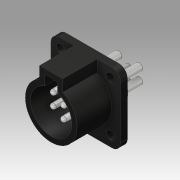
# Autodesk Inventor part: 6pin
Saved by Autodesk Inventor 2019.3 (Build 233278000, 278)
## iProperties
Created: 2019-05-28
Part Number: 6pin
Material: Generic
Document SubType Name: Modeling
Designer: Dave
Density: 1 g/cm^3
Appearance: Default
Author: Dave
Autodesk Inventor part; units mm, degrees
ref_plane "YZ Plane" through (0, 0, 0) normal (1, 0, 0) x (0, 1, 0)
ref_plane "XZ Plane" through (0, 0, 0) normal (0, 1, 0) x (-1, 0, 0)
ref_plane "XY Plane" through (0, 0, 0) normal (0, 0, 1) x (1, 0, 0)
sketch "Sketch1" plane through (0, 0, 0) normal (0, 0, 1) x (1, 0, 0)
  line L0 (2.5, 0) -> (17.7, 0)
  line L1 (20.2, 2.5) -> (20.2, 17.7)
  line L2 (17.7, 20.2) -> (2.5, 20.2)
  line L3 (0, 17.7) -> (0, 2.5)
  circle A0 centre (2.85, 17.35) radius 1.25
  circle A1 centre (17.35, 17.35) radius 1.25
  circle A2 centre (17.35, 2.85) radius 1.25
  circle A3 centre (2.85, 2.85) radius 1.25
  arc A4 (2.5, 20.2) -> (0, 17.7) centre (2.5, 17.7) ccw
  arc A5 (20.2, 17.7) -> (17.7, 20.2) centre (17.7, 17.7) ccw
  arc A6 (17.7, 0) -> (20.2, 2.5) centre (17.7, 2.5) ccw
  arc A7 (0, 2.5) -> (2.5, 0) centre (2.5, 2.5) ccw
  circle A8 centre (10.1, 10.1) radius 10.253 construction
  arc A9 (6.75, 16.8103) -> (13.45, 16.8103) centre (10.1, 10.1) ccw
  line L4 (6.75, 20.2) -> (13.45, 20.2)
  line L5 (13.45, 20.2) -> (13.45, 16.8103)
  line L6 (6.75, 16.8103) -> (6.75, 20.2)
  point P0 (0, 0)
  point P1 (20.2, 20.2)
  point P2 (20.2, 0)
  point P3 (0, 20.2)
  point P4 (20.2, 10.1)
  point P5 (10.1, 20.2)
  point P6 (10.1, 16.8103)
  dimension "d0" = 20.2
  dimension "d1" = 20.2
  dimension "d2" = 2.5
  dimension "d3" = 17
  dimension "d4" = 17
  dimension "d5" = 2.5
  dimension "d6" = 15
  dimension "d7" = 17.6
  dimension "d8" = 6.7
  dimension "d9" = 3.35
  constraints: 14 end point, 13 point on circle, 10 centre point, 8 point on line, 8 tangent, 6 equal radius, 4 vertical alignment, 3 horizontal alignment, 3 parallel, 2 horizontal, 2 midpoint, 2 perpendicular, 1 coincident
  measures "d0" distance of point (20.2, 20.2) point (0, 20.2)
  measures "d1" distance of point (20.2, 0) point (20.2, 20.2)
  measures "d2" diameter of A0
  measures "d5" radius of A4
  measures "d6" diameter of A9
  measures "d8" distance between parallel lines of L5 L6
  measures "d9" distance from line of point (10.1, 20.2) L5
extrude "Extrusion1" add sketch "Sketch1" along normal blind 2
sketch "Sketch2" plane through (0, 0, 2) normal (0, 0, 1) x (1, 0, 0)
  line L0 (17.7, 20.2) -> (2.5, 20.2) projected
  circle A0 centre (2.85, 2.85) radius 1.25 projected
  circle A1 centre (17.35, 2.85) radius 1.25 projected
  circle A2 centre (17.35, 17.35) radius 1.25 projected
  circle A3 centre (2.85, 17.35) radius 1.25 projected
  line L1 (17.7, 20.2) -> (2.5, 20.2) projected
  arc A4 (2.5, 20.2) -> (0, 17.7) centre (2.5, 17.7) ccw projected
  line L2 (0, 17.7) -> (0, 2.5) projected
  arc A5 (0, 2.5) -> (2.5, 0) centre (2.5, 2.5) ccw projected
  line L3 (2.5, 0) -> (17.7, 0) projected
  arc A6 (17.7, 0) -> (20.2, 2.5) centre (17.7, 2.5) ccw projected
  line L4 (20.2, 2.5) -> (20.2, 17.7) projected
  arc A7 (20.2, 17.7) -> (17.7, 20.2) centre (17.7, 17.7) ccw projected
  arc A8 (6.75, 16.8103) -> (13.45, 16.8103) centre (10.1, 10.1) ccw
  line L5 (6.75, 20.2) -> (13.45, 20.2)
  line L6 (13.45, 20.2) -> (13.45, 16.8103)
  line L7 (6.75, 16.8103) -> (6.75, 20.2)
  line L8 (11.95, 15.8077) -> (11.95, 18.7)
  line L9 (11.95, 18.7) -> (8.25, 18.7)
  line L10 (8.25, 18.7) -> (8.25, 15.8077)
  arc A9 (8.25, 15.8077) -> (11.95, 15.8077) centre (10.1, 10.1) ccw
  point P0 (0, 0)
  point P1 (0, 10.1)
  point P2 (10.1, 20.2)
  point P3 (10.1, 20.2)
  point P4 (10.1, 20.2)
  dimension "d12" = 15
  dimension "d13" = 6.7
  dimension "d14" = 10.1
  dimension "d15" = 1.5
  constraints: 12 end point, 4 midpoint, 4 point on circle, 2 centre point, 2 parallel, 2 perpendicular, 1 coincident, 1 horizontal, 1 horizontal alignment, 1 vertical alignment, 3 other
  measures "d12" diameter of A8
  measures "d13" distance between parallel lines of L6 L7
  measures "d14" distance of A8.centre point (10.1, 20.2)
  measures "d15" radial gap between concentric circles of A8 A9
extrude "Extrusion2" add sketch "Sketch2" along normal blind 10 contours L6 A8 L7 L0
sketch "Sketch3" plane through (0, 0, 2) normal (0, 0, 1) x (1, 0, 0)
  circle A0 centre (10.1, 13.6) radius 0.75
  arc A1 (8.25, 15.8077) -> (11.95, 15.8077) centre (10.1, 10.1) ccw projected
  circle A2 centre (13.1311, 11.85) radius 0.75
  circle A3 centre (13.1311, 8.35) radius 0.75
  circle A4 centre (10.1, 6.6) radius 0.75
  circle A5 centre (7.0689, 8.35) radius 0.75
  circle A6 centre (7.0689, 11.85) radius 0.75
  circle A7 centre (10.1, 10.1) radius 0.75
  point P0 (0, 0)
  dimension "d20" = 360
  dimension "d22" = 1.5
  dimension "d23" = 3.5
  constraints: 7 centre point, 1 coincident, 1 equal radius, 1 vertical alignment, 13 other
  measures "d22" diameter of A0
  measures "d23" distance of A0.centre A1.centre
extrude "Extrusion3" add sketch "Sketch3" along normal blind 7 contours A2 | A3 | A4 | A5 | A6 | A7
fillet "Fillet1" radius 0.75 6 edges at (6.3189, 11.85, 9) (9.35, 10.1, 9) (12.3811, 11.85, 9) (12.3811, 8.35, 9) (9.35, 6.6, 9) (6.3189, 8.35, 9)
sketch "Sketch4" plane through (0, 0, 0) normal (0, 0, -1) x (-1, 0, 0)
  circle A0 centre (-7.0689, 11.85) radius 0.75 projected
  circle A1 centre (-7.0689, 8.35) radius 0.75 projected
  circle A2 centre (-10.1, 6.6) radius 0.75 projected
  circle A3 centre (-10.1, 10.1) radius 0.75 projected
  circle A4 centre (-13.1311, 11.85) radius 0.75 projected
  circle A5 centre (-13.1311, 8.35) radius 0.75 projected
  circle A6 centre (-10.1, 10.1) radius 6.25
  line L0 (-14.162, 14.85) -> (-6.038, 14.85)
  line L1 (-11.1, 14.85) -> (-9.1, 14.85)
  line L2 (-9.1, 14.85) -> (-9.1, 12.35)
  line L3 (-9.1, 12.35) -> (-11.1, 12.35)
  line L4 (-11.1, 12.35) -> (-11.1, 14.85)
  point P0 (0, 0)
  point P1 (-10.1, 12.35)
  dimension "d27" = 12.5
  dimension "d28" = 11
  dimension "d29" = 2
  dimension "d30" = 2.5
  constraints: 10 end point, 2 horizontal, 2 parallel, 2 point on circle, 1 centre point, 1 coincident, 1 midpoint, 1 perpendicular, 1 point on line, 1 vertical alignment
  measures "d27" diameter of A6
  measures "d29" distance of L2.end L3.end
  measures "d30" distance between parallel lines of L3 L0
extrude "Extrusion4" add sketch "Sketch4" along normal blind 4 contours A0 | A1 | A2 | A3 | A4 | A5 | A6 L0 L4 L3 L2
sketch "Sketch5" plane through (0, 0, -4) normal (0, 0, -1) x (-1, 0, 0)
  circle A0 centre (-7.0689, 11.85) radius 0.75 projected
  circle A1 centre (-7.0689, 8.35) radius 0.75 projected
  circle A2 centre (-10.1, 10.1) radius 0.75 projected
  circle A3 centre (-13.1311, 11.85) radius 0.75 projected
  circle A4 centre (-13.1311, 8.35) radius 0.75 projected
  circle A5 centre (-10.1, 6.6) radius 0.75 projected
  circle A6 centre (-13.1311, 11.85) radius 1
  circle A7 centre (-13.1311, 8.35) radius 1
  circle A8 centre (-10.1, 10.1) radius 1
  circle A9 centre (-7.0689, 11.85) radius 1
  circle A10 centre (-7.0689, 8.35) radius 1
  circle A11 centre (-10.1, 6.6) radius 1
  point P0 (0, 0)
  dimension "d33" = 2
  constraints: 6 centre point, 6 coincident, 5 equal radius
  measures "d33" diameter of A6
extrude "Extrusion5" add sketch "Sketch5" along normal blind 6.5 contours A0 | A1 | A2 | A3 | A4 | A5 | A6 | A7 | A8 | A9 | A10 | A11
body "Solid1"
